Autodesk Fusion 360 part; units mm, degrees
note: some values were not read from the file. Set by a fixed rule: which sketch regions a step uses.
(part 2 of 5)
  line L811 (-126.9006, -75.4218) -> (-126.864, -75.6319)
  line L812 (-162.0421, -65.6576) -> (-162.1957, -65.5957)
  line L813 (-120.3905, -67.7689) -> (-120.173, -67.7759)
  line L814 (-90.103, -81.6973) -> (-90.112, -81.5125)
  line L815 (-65.5702, -65.5161) -> (-65.6778, -65.5555)
  line L816 (-93.5695, -76.6003) -> (-93.6281, -76.5038)
  line L817 (-126.8138, -65.8554) -> (-126.9169, -65.9479)
  line L818 (-87.0368, -78.1332) -> (-87.1608, -78.2349)
  line L819 (-140.2391, -65.691) -> (-140.3446, -65.6405)
  line L820 (-89.961, -66.5581) -> (-89.912, -66.407)
  line L821 (-115.4217, -76.295) -> (-115.4379, -76.172)
  line L822 (-129.347, -82.0733) -> (-129.353, -81.9536)
  line L823 (-50.3698, -71.3623) -> (-50.4116, -70.9586)
  line L824 (-93.7711, -77.986) -> (-93.6955, -77.9029)
  line L825 (-89.7734, -77.8951) -> (-89.8498, -77.7607)
  line L826 (-46.8782, -83.1526) -> (-46.7759, -83.1033)
  line L827 (-92.8846, -67.1853) -> (-92.9022, -67.0198)
  line L828 (-61.2627, -71.0913) -> (-61.2289, -70.9062)
  line L829 (-87.3025, -65.7007) -> (-87.1608, -65.7896)
  line L830 (-142.5953, -66.3913) -> (-142.6631, -66.5377)
  line L831 (-55.4106, -69.1495) -> (-55.2872, -69.243)
  line L832 (-103.1429, -65.6707) -> (-103.256, -65.7012)
  line L833 (-165.9299, -78.5695) -> (-165.7921, -78.5402)
  line L834 (-94.4542, -65.5719) -> (-94.5983, -65.5659)
  line L835 (-68.7045, -81.1031) -> (-68.801, -81.0445)
  line L836 (-169.2879, -78.2018) -> (-169.1558, -78.3005)
  line L837 (-123.2797, -75.1463) -> (-123.3556, -75.0225)
  line L838 (-76.8438, -76.0271) -> (-76.9461, -75.9778)
  line L839 (-55.8191, -68.9094) -> (-55.6766, -68.9828)
  line L840 (-62.1343, -82.9148) -> (-61.9869, -82.8077)
  line L841 (-80.9243, -80.5547) -> (-80.9006, -80.7493)
  line L842 (-121.6721, -67.9822) -> (-121.3798, -67.8915)
  line L843 (-76.9461, -75.9778) -> (-77.0536, -75.9384)
  line L844 (-163.1, -65.4919) -> (-163.2831, -65.5128)
  line L845 (-123.185, -75.2544) -> (-123.2797, -75.1463)
  line L846 (-101.2359, -66.5385) -> (-101.3094, -66.4135)
  line L847 (-120.0878, -75.693) -> (-120.2483, -75.693)
  line L848 (-116.4755, -75.1533) -> (-116.6326, -75.1503)
  line L849 (-87.0272, -82.7907) -> (-87.1556, -82.9073)
  line L850 (-53.6624, -82.7225) -> (-53.5344, -82.8302)
  line L851 (-121.4581, -71.9616) -> (-121.4203, -72.1465)
  line L852 (-133.3978, -83.1133) -> (-133.2339, -83.1617)
  line L853 (-132.6154, -83.2188) -> (-132.4975, -83.2377)
  line L854 (-141.2619, -78.1855) -> (-141.1327, -78.275)
  line L855 (-116.8006, -75.1659) -> (-120.0878, -75.693)
  line L856 (-169.912, -76.8783) -> (-169.903, -77.0537)
  line L857 (-123.4458, -74.7233) -> (-123.4576, -74.5459)
  line L858 (-121.3798, -67.8915) -> (-121.0683, -67.8246)
  line L859 (-120.6654, -78.2888) -> (-119.8307, -78.2988)
  line L860 (-119.8307, -78.2988) -> (-116.8014, -77.8018)
  line L861 (-134.2971, -66.4674) -> (-134.3507, -66.6361)
  line L862 (-111.0523, -65.5725) -> (-111.1974, -65.591)
  line L863 (-61.084, -70.3947) -> (-61.0214, -70.2386)
  line L864 (-130.9576, -67.0124) -> (-130.9813, -66.8178)
  line L865 (-142.5144, -66.252) -> (-142.5953, -66.3913)
  line L866 (-60.7916, -69.813) -> (-60.7012, -69.6851)
  line L867 (-59.2767, -68.7288) -> (-59.1098, -68.6816)
  line L868 (-94.7298, -65.5709) -> (-94.8598, -65.586)
  line L869 (-94.5986, -75.988) -> (-95.8873, -75.988)
  line L870 (-133.8257, -82.8864) -> (-133.6942, -82.9756)
  line L871 (-71.4648, -83.217) -> (-71.343, -83.2371)
  line L872 (-51.3135, -68.2591) -> (-51.4937, -67.9865)
  line L873 (-78.0556, -65.7513) -> (-78.1872, -65.6622)
  line L874 (-52.6036, -66.8344) -> (-52.8657, -66.6454)
  line L875 (-50.9966, -68.8468) -> (-51.1477, -68.5458)
  line L876 (-109.6365, -66.1302) -> (-109.7282, -66.0365)
  line L877 (-118.54, -68.7717) -> (-118.4981, -68.9082)
  line L878 (-59.8834, -68.9828) -> (-59.741, -68.9094)
  line L879 (-87.1608, -78.2349) -> (-87.3025, -78.3238)
  line L880 (-156.5375, -68.4558) -> (-156.4497, -68.5385)
  line L881 (-102.906, -65.6294) -> (-103.0505, -65.6498)
  line L882 (-89.4549, -82.9073) -> (-89.5832, -82.7907)
  line L883 (-61.5365, -82.243) -> (-61.4612, -82.0706)
  line L884 (-88.063, -78.5303) -> (-88.3059, -78.5393)
  line L885 (-90.037, -76.9765) -> (-90.042, -76.8042)
  line L886 (-141.3194, -65.4941) -> (-141.485, -65.5212)
  line L887 (-54.3644, -65.9031) -> (-54.7002, -65.7945)
  line L888 (-140.0758, -78.5266) -> (-139.8899, -78.489)
  line L889 (-110.6466, -65.5866) -> (-110.7765, -65.5715)
  line L890 (-126.9296, -74.973) -> (-126.9226, -75.2022)
  line L891 (-122.6439, -75.5491) -> (-122.801, -75.494)
  line L892 (-80.3369, -81.7452) -> (-80.2054, -81.8343)
  line L893 (-89.1489, -65.6257) -> (-88.9694, -65.5656)
  line L894 (-50.3366, -80.9037) -> (-50.3366, -72.2147)
  line L895 (-108.0032, -78.1266) -> (-107.8316, -78.1881)
  line L896 (-51.6881, -67.7282) -> (-51.8966, -67.4839)
  line L897 (-160.6206, -76.2253) -> (-160.7403, -76.2193)
  line L898 (-76.5741, -76.2287) -> (-76.6572, -76.1531)
  line L899 (-76.4986, -76.3118) -> (-76.5741, -76.2287)
  line L900 (-87.1556, -80.1182) -> (-87.0272, -80.2348)
  line L901 (-76.2839, -76.7083) -> (-76.3233, -76.6007)
  line L902 (-56.6229, -68.6408) -> (-56.4502, -68.6816)
  line L903 (-89.3159, -80.0143) -> (-89.1669, -79.9239)
  line L904 (-68.2121, -82.3098) -> (-68.1943, -82.1936)
  line L905 (-163.5051, -78.4641) -> (-163.3655, -78.4974)
  line L906 (-89.1669, -83.1019) -> (-89.3159, -83.0114)
  line L907 (-89.4507, -78.2349) -> (-89.5747, -78.1332)
  line L908 (-65.9667, -67.5363) -> (-65.8766, -67.6036)
  line L909 (-140.4165, -78.5316) -> (-140.2687, -78.5396)
  line L910 (-100.5686, -76.959) -> (-100.4851, -77.1166)
  line L911 (-111.7999, -65.8158) -> (-111.9405, -65.911)
  line L912 (-52.9126, -83.1337) -> (-52.7317, -83.1755)
  line L913 (-141.6874, -76.173) -> (-141.7635, -76.2923)
  line L914 (-95.4672, -65.8024) -> (-95.5765, -65.8721)
  line L915 (-77.8284, -65.9697) -> (-77.9359, -65.8538)
  line L916 (-86.9295, -66.005) -> (-86.8381, -66.1295)
  line L917 (-77.7337, -66.0989) -> (-77.8284, -65.9697)
  line L918 (-46.3046, -81.516) -> (-46.3632, -81.4195)
  line L919 (-87.941, -79.7427) -> (-87.7677, -79.7872)
  line L920 (-129.4881, -82.6312) -> (-129.4388, -82.5289)
  line L921 (-81.9787, -75.9472) -> (-82.1648, -75.9512)
  line L922 (-80.9323, -69.0045) -> (-80.9323, -75.9472)
  line L923 (-164.0956, -78.1584) -> (-163.9927, -78.2379)
  line L924 (-80.9323, -68.559) -> (-80.9323, -69.0045)
  line L925 (-77.1657, -78.2028) -> (-77.0536, -78.1739)
  line L926 (-108.6242, -77.7613) -> (-108.4802, -77.8696)
  line L927 (-93.6955, -77.9029) -> (-93.6281, -77.8128)
  line L928 (-89.8498, -66.2638) -> (-89.7734, -66.1295)
  line L929 (-102.7483, -65.6214) -> (-102.7533, -65.6214)
  line L930 (-77.2819, -78.2205) -> (-77.1657, -78.2028)
  line L931 (-77.4016, -78.2265) -> (-77.2819, -78.2205)
  line L932 (-88.3054, -79.7063) -> (-88.1205, -79.7153)
  line L933 (-52.3545, -67.0371) -> (-52.6036, -66.8344)
  line L934 (-72.1359, -83.085) -> (-71.9818, -83.1371)
  line L935 (-142.7171, -66.6901) -> (-142.7566, -66.8474)
  line L936 (-116.0697, -75.2646) -> (-116.1941, -75.2121)
  line L937 (-121.0683, -67.8246) -> (-120.7384, -67.7832)
  line L938 (-86.5074, -81.6973) -> (-86.5348, -81.8768)
  line L939 (-46.2553, -81.6183) -> (-46.3046, -81.516)
  line L940 (-78.1872, -65.6622) -> (-78.33, -65.5866)
  line L941 (-80.9323, -67.1493) -> (-80.9323, -68.559)
  line L942 (-68.4557, -82.8183) -> (-68.3883, -82.7282)
  line L943 (-77.6522, -66.2413) -> (-77.7337, -66.0989)
  line L944 (-106.2087, -78.1313) -> (-106.0461, -78.0602)
  line L945 (-61.8395, -66.1717) -> (-62.1152, -66.3088)
  line L946 (-69.632, -67.0129) -> (-69.6557, -66.8183)
  line L947 (-68.3883, -82.7282) -> (-68.3296, -82.6317)
  line L948 (-102.1409, -65.739) -> (-102.2516, -65.7009)
  line L949 (-141.3833, -78.0849) -> (-141.2619, -78.1855)
  line L950 (-62.9317, -66.2857) -> (-62.9711, -66.1782)
  line L951 (-106.5499, -78.2376) -> (-106.3768, -78.1906)
  line L952 (-160.2848, -78.4671) -> (-160.1826, -78.4179)
  line L953 (-160.5044, -76.243) -> (-160.6206, -76.2253)
  line L954 (-82.7955, -76.0449) -> (-82.9243, -76.0896)
  line L955 (-160.3923, -76.2718) -> (-160.5044, -76.243)
  line L956 (-164.4833, -77.6255) -> (-164.4235, -77.7499)
  line L957 (-54.237, -71.9056) -> (-54.237, -81.2746)
  line L958 (-160.3923, -78.5064) -> (-160.2848, -78.4671)
  line L959 (-82.9243, -76.0896) -> (-83.0413, -76.1434)
  line L960 (-160.2848, -76.3111) -> (-160.3923, -76.2718)
  line L961 (-130.3974, -80.9088) -> (-130.5171, -80.9028)
  line L962 (-112.6217, -67.1857) -> (-112.6227, -67.3536)
  line L963 (-86.8066, -80.5021) -> (-86.7161, -80.6511)
  line L964 (-54.241, -71.6908) -> (-54.237, -71.9056)
  line L965 (-90.0756, -81.1482) -> (-90.0311, -80.975)
  line L966 (-60.9517, -65.8277) -> (-61.2576, -65.9312)
  line L967 (-87.6422, -65.5656) -> (-87.4627, -65.6257)
  line L968 (-77.5844, -81.0996) -> (-77.5308, -80.931)
  line L969 (-77.7337, -81.3976) -> (-77.6522, -81.2552)
  line L970 (-130.1691, -80.9553) -> (-130.2812, -80.9265)
  line L971 (-110.908, -65.5665) -> (-111.0523, -65.5725)
  line L972 (-66.3009, -67.089) -> (-66.2516, -67.1913)
  line L973 (-77.9359, -65.8538) -> (-78.0556, -65.7513)
  line L974 (-77.4602, -68.559) -> (-77.4602, -67.1493)
  line L975 (-160.0861, -78.3594) -> (-159.996, -78.2921)
  line L976 (-132.8771, -83.2173) -> (-132.6852, -83.2248)
  line L977 (-93.5666, -65.9106) -> (-93.7072, -65.8154)
  line L978 (-63.6988, -83.1888) -> (-63.4915, -83.2157)
  line L979 (-140.4577, -65.5959) -> (-140.5788, -65.5579)
  line L980 (-65.2215, -71.648) -> (-65.207, -71.7916)
  line L981 (-92.9826, -67.8593) -> (-92.9319, -67.6912)
  line L982 (-69.816, -66.3124) -> (-69.8975, -66.17)
  line L983 (-89.309, -65.7007) -> (-89.1489, -65.6257)
  line L984 (-46.1692, -82.1938) -> (-46.1632, -82.0741)
  line L985 (-94.479, -75.994) -> (-94.5986, -75.988)
  line L986 (-66.1255, -65.8894) -> (-66.1929, -65.9795)
  line L987 (-46.187, -81.8381) -> (-46.2159, -81.7259)
  line L988 (-94.1431, -76.0799) -> (-94.2506, -76.0405)
  line L989 (-133.9455, -65.9244) -> (-134.053, -66.0402)
  line L990 (-88.3059, -65.4852) -> (-88.063, -65.4942)
  line L991 (-140.8562, -78.4181) -> (-140.7116, -78.4701)
  line L992 (-135.39, -73.3534) -> (-135.3726, -73.1817)
  line L993 (-68.6144, -81.1705) -> (-68.7045, -81.1031)
  line L994 (-142.6631, -66.5377) -> (-142.7171, -66.6901)
  line L995 (-131.3176, -66.0402) -> (-131.425, -65.9244)
  line L996 (-141.9093, -76.9708) -> (-141.8993, -77.1333)
  line L997 (-69.6557, -66.8183) -> (-69.6946, -66.6366)
  line L998 (-106.0461, -78.0602) -> (-105.8898, -77.9776)
  line L999 (-50.7395, -69.4922) -> (-50.8605, -69.1623)
  line L1000 (-129.9593, -83.1025) -> (-129.8628, -83.0439)
  line L1001 (-134.053, -82.6678) -> (-133.9455, -82.7838)
  line L1002 (-50.6339, -69.8368) -> (-50.7395, -69.4922)
  line L1003 (-77.1657, -75.9096) -> (-77.2819, -75.8919)
  line L1004 (-129.6141, -82.8178) -> (-129.5467, -82.7277)
  line L1005 (-105.4645, -77.6658) -> (-105.3395, -77.542)
  line L1006 (-93.8589, -65.7335) -> (-94.0212, -65.666)
  line L1007 (-89.7734, -66.1295) -> (-89.682, -66.005)
  line L1008 (-54.1178, -82.0155) -> (-54.0527, -82.1779)
  line L1009 (-86.6505, -77.4665) -> (-86.6995, -77.6175)
  line L1010 (-107.6547, -78.2368) -> (-107.4733, -78.2722)
  line L1011 (-80.9006, -80.7493) -> (-80.8617, -80.931)
  line L1012 (-63.3951, -65.6634) -> (-63.4916, -65.6048)
  line L1013 (-61.5536, -66.0458) -> (-61.8395, -66.1717)
  line L1014 (-80.8081, -66.3968) -> (-80.8617, -66.5655)
  line L1015 (-131.819, -65.6573) -> (-131.9726, -65.5954)
  line L1016 (-65.1882, -81.6928) -> (-65.1452, -81.887)
  line L1017 (-89.682, -66.005) -> (-89.5747, -65.8914)
  line L1018 (-131.2229, -66.1694) -> (-131.3176, -66.0402)
  line L1019 (-82.3396, -78.2162) -> (-82.1648, -78.2274)
  line L1020 (-82.6551, -76.009) -> (-82.7955, -76.0449)
  line L1021 (-160.7403, -78.5589) -> (-160.6206, -78.5529)
  line L1022 (-165.2902, -78.3193) -> (-165.1793, -78.2406)
  line L1023 (-164.5745, -77.3505) -> (-164.5337, -77.4924)
  line L1024 (-160.6206, -78.5529) -> (-160.5044, -78.5352)
  line L1025 (-163.6379, -78.4215) -> (-163.5051, -78.4641)
  line L1026 (-102.0887, -65.7551) -> (-102.1409, -65.739)
  line L1027 (-129.4388, -82.5289) -> (-129.3995, -82.4213)
  line L1028 (-78.1873, -81.8343) -> (-78.0558, -81.7452)
  line L1029 (-79.1963, -65.4138) -> (-79.3881, -65.4208)
  line L1030 (-79.3881, -65.4208) -> (-79.5712, -65.4417)
  line L1031 (-80.0624, -65.5866) -> (-80.2052, -65.6622)
  line L1032 (-77.0536, -78.1739) -> (-76.9461, -78.1345)
  line L1033 (-76.9461, -78.1345) -> (-76.8438, -78.0852)
  line L1034 (-80.4566, -81.6427) -> (-80.3369, -81.7452)
  line L1035 (-87.0368, -65.8914) -> (-86.9295, -66.005)
  line L1036 (-82.7955, -78.134) -> (-82.6551, -78.1698)
  line L1037 (-77.2819, -75.8919) -> (-77.4016, -75.8859)
  line L1038 (-142.4321, -68.291) -> (-138.8179, -73.1413)
  line L1039 (-133.0602, -65.5125) -> (-133.2339, -65.5471)
  line L1040 (-63.8136, -65.4873) -> (-63.9298, -65.4696)
  line L1041 (-117.4702, -65.7305) -> (-117.6443, -65.6736)
  line L1042 (-78.6478, -82.0202) -> (-78.4838, -81.9719)
  line L1043 (-66.3928, -66.6336) -> (-66.3868, -66.7532)
  line L1044 (-53.4283, -66.3082) -> (-53.7283, -66.1599)
  line L1045 (-93.6281, -77.8128) -> (-93.5695, -77.7163)
  line L1046 (-68.2409, -82.4219) -> (-68.2121, -82.3098)
  line L1047 (-139.3769, -78.2514) -> (-139.2218, -78.1381)
  line L1048 (-76.3726, -76.4984) -> (-76.4312, -76.4019)
  line L1049 (-142.5381, -68.1262) -> (-142.4321, -68.291)
  line L1050 (-86.5888, -66.8796) -> (-86.5744, -67.0481)
  line L1051 (-86.9106, -80.3631) -> (-86.8066, -80.5021)
  line L1052 (-78.33, -65.5866) -> (-78.4836, -65.5246)
  line L1053 (-89.1669, -79.9239) -> (-89.0089, -79.8479)
  line L1054 (-52.1188, -67.2535) -> (-52.3545, -67.0371)
  line L1055 (-92.8991, -67.5221) -> (-92.8836, -67.3531)
  line L1056 (-78.4836, -65.5246) -> (-78.6475, -65.4763)
  line L1057 (-78.6475, -65.4763) -> (-78.8213, -65.4417)
  line L1058 (-77.5308, -66.5655) -> (-77.5844, -66.3968)
  line L1059 (-65.3418, -65.4696) -> (-65.458, -65.4873)
  line L1060 (-77.5844, -66.3968) -> (-77.6522, -66.2413)
  line L1061 (-100.6403, -76.7941) -> (-100.5686, -76.959)
  line L1062 (-61.1395, -70.5579) -> (-61.084, -70.3947)
  line L1063 (-87.6422, -78.4589) -> (-87.842, -78.5031)
  line L1064 (-71.6462, -83.2032) -> (-71.4648, -83.217)
  line L1065 (-94.1649, -65.6216) -> (-94.3095, -65.5904)
  line L1066 (-65.207, -71.7916) -> (-65.2174, -72.0012)
  line L1067 (-140.708, -65.5271) -> (-140.8458, -65.5044)
  line L1068 (-131.9726, -65.5954) -> (-132.1365, -65.5471)
  line L1069 (-134.2971, -82.2404) -> (-134.2293, -82.396)
  line L1070 (-108.8856, -77.5138) -> (-108.7595, -77.6426)
  line L1071 (-64.5603, -82.8077) -> (-64.4129, -82.9148)
  line L1072 (-61.9869, -82.8077) -> (-61.8529, -82.6864)
  line L1073 (-93.4342, -77.2781) -> (-93.4282, -77.1585)
  line L1074 (-89.4507, -65.7896) -> (-89.309, -65.7007)
  line L1075 (-50.8605, -69.1623) -> (-50.9966, -68.8468)
  line L1076 (-77.4602, -78.2305) -> (-77.4602, -78.2265)
  line L1077 (-87.1556, -82.9073) -> (-87.2947, -83.0114)
  line L1078 (-56.4502, -68.6816) -> (-56.2833, -68.7288)
  line L1079 (-66.3691, -66.8694) -> (-66.3403, -66.9815)
  line L1080 (-141.5971, -77.8536) -> (-141.4955, -77.9741)
  line L1081 (-63.2219, -65.8063) -> (-63.305, -65.7308)
  line L1082 (-79.0043, -65.4208) -> (-79.1963, -65.4138)
  line L1083 (-76.6572, -76.1531) -> (-76.7473, -76.0857)
  line L1084 (-80.2052, -65.6622) -> (-80.3368, -65.7513)
  line L1085 (-100.045, -77.6636) -> (-99.9116, -77.7774)
  line L1086 (-76.7473, -78.0266) -> (-76.6572, -77.9592)
  line L1087 (-77.4919, -80.7493) -> (-77.4682, -80.5547)
  line L1088 (-63.1464, -65.8894) -> (-63.2219, -65.8063)
  line L1089 (-77.4602, -67.1493) -> (-77.4682, -66.9418)
  line L1090 (-78.0558, -81.7452) -> (-77.936, -81.6427)
  line L1091 (-92.9319, -67.6912) -> (-92.8991, -67.5221)
  line L1092 (-108.169, -78.0527) -> (-108.0032, -78.1266)
  line L1093 (-70.9852, -65.5129) -> (-71.1683, -65.492)
  line L1094 (-46.187, -82.31) -> (-46.1692, -82.1938)
  line L1095 (-65.2144, -81.4884) -> (-65.1882, -81.6928)
  line L1096 (-141.8708, -76.5779) -> (-141.8993, -76.7576)
  line L1097 (-99.1359, -78.1876) -> (-98.9634, -78.2348)
  line L1098 (-68.5313, -82.9014) -> (-68.4557, -82.8183)
  line L1099 (-134.4213, -73.5926) -> (-134.4213, -81.4877)
  line L1100 (-164.6721, -77.6095) -> (-164.6183, -77.4824)
  line L1101 (-81.9787, -78.2305) -> (-80.9323, -78.2305)
  line L1102 (-164.1904, -78.0698) -> (-164.0956, -78.1584)
  line L1103 (-66.3403, -66.9815) -> (-66.3009, -67.089)
  line L1104 (-69.3591, -83.2441) -> (-69.2394, -83.2381)
  line L1105 (-132.8771, -65.4916) -> (-133.0602, -65.5125)
  line L1106 (-51.4937, -67.9865) -> (-51.6881, -67.7282)
  line L1107 (-79.7449, -65.4763) -> (-79.9088, -65.5246)
  line L1108 (-52.8657, -66.6454) -> (-53.1407, -66.4701)
  line L1109 (-86.64, -80.809) -> (-86.5793, -80.975)
  line L1110 (-66.1929, -65.9795) -> (-66.2516, -66.076)
  line L1111 (-65.6778, -65.5555) -> (-65.7801, -65.6048)
  line L1112 (-66.0499, -65.8063) -> (-66.1255, -65.8894)
  line L1113 (-58.167, -65.3954) -> (-58.5464, -65.4115)
  line L1114 (-69.3591, -80.9033) -> (-69.624, -80.9033)
  line L1115 (-77.4682, -66.9418) -> (-77.4919, -66.7472)
  line L1116 (-80.7403, -66.2413) -> (-80.8081, -66.3968)
  line L1117 (-140.997, -78.3528) -> (-140.8562, -78.4181)
  line L1118 (-106.3768, -78.1906) -> (-106.2087, -78.1313)
  line L1119 (-166.4853, -75.6143) -> (-168.1963, -75.6143)
  line L1120 (-123.3556, -75.0225) -> (-123.4114, -74.8818)
  line L1121 (-86.5744, -76.9765) -> (-86.5888, -77.145)
  line L1122 (-77.4602, -78.2265) -> (-77.4016, -78.2265)
  line L1123 (-73.089, -81.689) -> (-73.0668, -81.8773)
  line L1124 (-71.7351, -65.5129) -> (-71.9088, -65.5475)
  line L1125 (-94.5983, -65.5659) -> (-94.7298, -65.5709)
  line L1126 (-169.5204, -77.9693) -> (-169.4097, -78.0911)
  line L1127 (-89.5832, -80.2348) -> (-89.4549, -80.1182)
  line L1128 (-141.825, -77.4421) -> (-141.7632, -77.5869)
  line L1129 (-68.2803, -81.618) -> (-68.3296, -81.5157)
  line L1130 (-80.0626, -81.9099) -> (-79.909, -81.9719)
  line L1131 (-59.9762, -65.5837) -> (-60.3108, -65.654)
  line L1132 (-63.9298, -65.4696) -> (-64.0494, -65.4636)
  line L1133 (-88.4902, -83.3107) -> (-88.6697, -83.2833)
  line L1134 (-62.6352, -66.6169) -> (-62.8792, -66.7881)
  line L1135 (-77.6522, -81.2552) -> (-77.5844, -81.0996)
  line L1136 (-88.6697, -79.7427) -> (-88.4902, -79.7153)
  line L1137 (-71.8185, -83.1765) -> (-71.6462, -83.2032)
  line L1138 (-141.6868, -77.7243) -> (-141.5971, -77.8536)
  line L1139 (-90.042, -67.2203) -> (-90.037, -67.0481)
  line L1140 (-131.5448, -65.8219) -> (-131.6763, -65.7328)
  line L1141 (-53.395, -82.9256) -> (-53.2446, -83.0083)
  line L1142 (-141.485, -65.5212) -> (-141.644, -65.5652)
  line L1143 (-134.053, -66.0402) -> (-134.1478, -66.1694)
  line L1144 (-136.2972, -70.9305) -> (-139.5794, -66.2933)
  line L1145 (-54.229, -81.4727) -> (-54.2064, -81.6625)
  line L1146 (-96.1018, -66.4544) -> (-96.1626, -66.5764)
  line L1147 (-123.4114, -74.8818) -> (-123.4458, -74.7233)
  line L1148 (-53.7283, -66.1599) -> (-54.0404, -66.0248)
  line L1149 (-121.0588, -72.7204) -> (-120.9345, -72.8083)
  line L1150 (-71.2172, -83.2441) -> (-69.3591, -83.2441)
  line L1151 (-101.5617, -66.1074) -> (-101.65, -66.0281)
  line L1152 (-139.965, -65.8704) -> (-140.1409, -65.7466)
  line L1153 (-135.4061, -72.608) -> (-135.4516, -72.4184)
  line L1154 (-80.9323, -75.9472) -> (-81.9787, -75.9472)
  line L1155 (-141.9397, -65.6991) -> (-142.0749, -65.7869)
  line L1156 (-107.0214, -73.0608) -> (-109.2926, -66.7055)
  line L1157 (-93.5202, -76.7026) -> (-93.5695, -76.6003)
  line L1158 (-72.6504, -82.7506) -> (-72.538, -82.853)
  line L1159 (-65.9667, -65.7308) -> (-66.0499, -65.8063)
  line L1160 (-93.7072, -65.8154) -> (-93.8589, -65.7335)
  line L1161 (-132.1365, -65.5471) -> (-132.3103, -65.5125)
  line L1162 (-112.1863, -66.137) -> (-112.2905, -66.2655)
  line L1163 (-61.3325, -81.4884) -> (-61.3235, -81.2746)
  line L1164 (-64.8142, -82.5514) -> (-64.6942, -82.6864)
  line L1165 (-72.9802, -82.2175) -> (-72.9166, -82.3692)
  line L1166 (-140.7116, -78.4701) -> (-140.5646, -78.5082)
  line L1167 (-86.9295, -78.0196) -> (-87.0368, -78.1332)
  line L1168 (-133.8257, -65.8219) -> (-133.9455, -65.9244)
  line L1169 (-61.2289, -70.9062) -> (-61.1878, -70.7284)
  line L1170 (-86.5694, -67.2203) -> (-86.5694, -76.8042)
  line L1171 (-69.1231, -80.927) -> (-69.2394, -80.9093)
  line L1172 (-72.904, -66.3124) -> (-72.9718, -66.468)
  line L1173 (-89.1489, -78.3988) -> (-89.309, -78.3238)
  line L1174 (-135.641, -74.1334) -> (-135.54, -73.9208)
  line L1175 (-133.5514, -83.0512) -> (-133.3978, -83.1133)
  line L1176 (-72.3691, -65.7333) -> (-72.5006, -65.8224)
  line L1177 (-65.0105, -82.243) -> (-64.9198, -82.4034)
  line L1178 (-98.9634, -78.2348) -> (-98.7865, -78.2694)
  line L1179 (-52.2486, -83.2445) -> (-47.3337, -83.2445)
  line L1180 (-120.8032, -72.878) -> (-120.6684, -72.9315)
  line L1181 (-72.4145, -82.9429) -> (-72.2803, -83.0202)
  line L1182 (-111.1974, -65.591) -> (-111.3423, -65.6222)
  line L1183 (-121.1729, -72.6123) -> (-121.0588, -72.7204)
  line L1184 (-76.2374, -77.1762) -> (-76.2314, -77.0566)
  line L1185 (-63.079, -65.9795) -> (-63.1464, -65.8894)
  line L1186 (-63.0204, -66.076) -> (-63.079, -65.9795)
  line L1187 (-46.6794, -81.1034) -> (-46.7759, -81.0448)
  line L1188 (-102.7551, -65.6214) -> (-102.7591, -65.6214)
  line L1189 (-70.8115, -65.5475) -> (-70.9852, -65.5129)
  line L1190 (-159.8374, -76.6449) -> (-159.9129, -76.5618)
  line L1191 (-68.6144, -82.9769) -> (-68.5313, -82.9014)
  line L1192 (-83.3896, -76.4563) -> (-83.4462, -76.5605)
  line L1193 (-82.1648, -75.9512) -> (-82.3396, -75.9626)
  line L1194 (-82.3396, -75.9626) -> (-82.5031, -75.9816)
  line L1195 (-131.6763, -65.7328) -> (-131.819, -65.6573)
  line L1196 (-129.8628, -83.0439) -> (-129.7727, -82.9765)
  line L1197 (-165.7921, -78.5402) -> (-165.6589, -78.5)
  line L1198 (-82.5031, -75.9816) -> (-82.6551, -76.009)
  line L1199 (-123.4038, -69.8118) -> (-123.3375, -69.5795)
  line L1200 (-93.5695, -77.7163) -> (-93.5202, -77.614)
  line L1201 (-138.8179, -73.1413) -> (-141.3861, -75.8284)
  line L1202 (-76.4312, -76.4019) -> (-76.4986, -76.3118)
  line L1203 (-115.8534, -75.4086) -> (-115.9561, -75.3306)
  line L1204 (-135.3666, -72.9978) -> (-135.3769, -72.8016)
  line L1205 (-139.6868, -66.1494) -> (-139.8145, -66.0066)
  line L1206 (-118.4726, -69.384) -> (-118.5, -69.5598)
  line L1207 (-62.3805, -66.4572) -> (-62.6352, -66.6169)
  line L1208 (-62.8792, -66.7881) -> (-62.8792, -66.6336)
  line L1209 (-63.5939, -65.5555) -> (-63.7014, -65.5161)
  line L1210 (-130.2812, -83.22) -> (-130.1691, -83.1912)
  line L1211 (-63.4916, -65.6048) -> (-63.5939, -65.5555)
  line L1212 (-162.5987, -78.5589) -> (-160.7403, -78.5589)
  line L1213 (-68.2803, -82.5294) -> (-68.2409, -82.4219)
  line L1214 (-162.72, -78.5529) -> (-162.5987, -78.5589)
  line L1215 (-159.996, -76.4863) -> (-160.0861, -76.419)
  line L1216 (-76.2374, -76.9369) -> (-76.2551, -76.8206)
  line L1217 (-68.3296, -81.5157) -> (-68.3883, -81.4192)
  line L1218 (-83.2396, -76.2797) -> (-83.3207, -76.3628)
  line L1219 (-69.9923, -66.0408) -> (-70.0998, -65.9249)
  line L1220 (-96.2143, -66.7049) -> (-98.4858, -73.0619)
  line L1221 (-71.9088, -65.5475) -> (-72.0727, -65.5958)
  line L1222 (-88.8429, -79.7872) -> (-88.6697, -79.7427)
  line L1223 (-159.7115, -76.8314) -> (-159.7701, -76.7349)
  line L1224 (-134.1478, -66.1694) -> (-134.2293, -66.3118)
  line L1225 (-83.4904, -76.6757) -> (-83.5221, -76.8021)
  line L1226 (-58.937, -68.6408) -> (-58.574, -68.5784)
  line L1227 (-101.65, -66.0281) -> (-101.743, -65.9554)
  line L1228 (-164.5337, -77.4924) -> (-164.4833, -77.6255)
  line L1229 (-159.7701, -76.7349) -> (-159.8374, -76.6449)
  line L1230 (-147.3075, -77.2905) -> (-147.0665, -77.0991)
  line L1231 (-78.4838, -81.9719) -> (-78.3302, -81.9099)
  line L1232 (-86.4984, -81.5125) -> (-86.5074, -81.6973)
  line L1233 (-83.4462, -76.5605) -> (-83.4904, -76.6757)
  line L1234 (-71.1683, -65.492) -> (-71.3602, -65.485)
  line L1235 (-139.8145, -66.0066) -> (-139.965, -65.8704)
  line L1236 (-76.5741, -77.8837) -> (-76.4986, -77.8006)
  line L1237 (-87.7677, -83.2388) -> (-87.941, -83.2833)
  line L1238 (-61.0214, -70.2386) -> (-60.9517, -70.0896)
  line L1239 (-139.5794, -66.2933) -> (-139.6868, -66.1494)
  line L1240 (-129.353, -81.9536) -> (-129.3707, -81.8373)
  line L1241 (-139.8899, -78.489) -> (-139.7112, -78.4291)
  line L1242 (-77.4919, -66.7472) -> (-77.5308, -66.5655)
  line L1243 (-54.539, -70.2386) -> (-54.4764, -70.3947)
  line L1244 (-57.3718, -68.5413) -> (-56.986, -68.5784)
  line L1245 (-46.5893, -81.1708) -> (-46.6794, -81.1034)
  line L1246 (-55.0473, -65.699) -> (-55.4058, -65.6166)
  line L1247 (-76.2314, -77.0566) -> (-76.2374, -76.9369)
  line L1248 (-93.4375, -66.0181) -> (-93.5666, -65.9106)
  line L1249 (-88.1205, -83.3107) -> (-88.3054, -83.3197)
  line L1250 (-77.4602, -80.3472) -> (-77.4602, -78.2305)
  line L1251 (-104.3427, -66.6878) -> (-107.0214, -73.0608)
  line L1252 (-53.1407, -66.4701) -> (-53.4283, -66.3082)
  line L1253 (-107.4733, -78.2722) -> (-107.288, -78.2938)
  line L1254 (-163.7636, -78.3695) -> (-163.6379, -78.4215)
  line L1255 (-63.7014, -65.5161) -> (-63.8136, -65.4873)
  line L1256 (-69.1231, -83.2204) -> (-69.0109, -83.1916)
  line L1257 (-119.8428, -73.0222) -> (-119.3494, -72.958)
  line L1258 (-163.882, -78.3083) -> (-163.7636, -78.3695)
  line L1259 (-87.6017, -79.8479) -> (-87.4437, -79.9239)
  line L1260 (-160.0861, -76.419) -> (-160.1826, -76.3604)
  line L1261 (-83.0413, -76.1434) -> (-83.1465, -76.2067)
  line L1262 (-70.3511, -65.7333) -> (-70.4939, -65.6578)
  line L1263 (-160.1826, -76.3604) -> (-160.2848, -76.3111)
  line L1264 (-66.3868, -66.514) -> (-66.3928, -66.6336)
  line L1265 (-95.2348, -65.6887) -> (-95.3531, -65.7412)
  line L1266 (-70.6475, -65.5958) -> (-70.8115, -65.5475)
  line L1267 (-159.9129, -76.5618) -> (-159.996, -76.4863)
  line L1268 (-83.3896, -77.7235) -> (-83.3207, -77.8168)
  line L1269 (-133.2339, -65.5471) -> (-133.3978, -65.5954)
  line L1270 (-83.1465, -76.2067) -> (-83.2396, -76.2797)
  line L1271 (-86.6139, -66.7159) -> (-86.5888, -66.8796)
  line L1272 (-163.3655, -78.4974) -> (-163.2193, -78.5212)
  line L1273 (-83.3207, -76.3628) -> (-83.3896, -76.4563)
  line L1274 (-98.3201, -78.293) -> (-98.1858, -78.3189)
  line L1275 (-112.5246, -67.8603) -> (-109.3525, -76.7362)
  line L1276 (-164.8891, -77.9561) -> (-164.808, -77.8468)
  line L1277 (-141.3861, -75.8284) -> (-141.5982, -76.0604)
  line L1278 (-150.0636, -68.4918) -> (-149.9234, -68.559)
  line L1279 (-105.2238, -77.4089) -> (-105.1182, -77.267)
  line L1280 (-161.6481, -65.9247) -> (-161.7678, -65.8222)
  line L1281 (-64.6942, -82.6864) -> (-64.5603, -82.8077)
  line L1282 (-102.7533, -65.6214) -> (-102.7543, -65.6214)
  line L1283 (-59.2792, -65.4759) -> (-59.6322, -65.5243)
  line L1284 (-72.8402, -82.5087) -> (-72.7513, -82.6359)
  line L1285 (-80.6588, -66.0989) -> (-80.7403, -66.2413)
  line L1286 (-110.5188, -65.6115) -> (-110.6466, -65.5866)
  line L1287 (-68.3296, -82.6317) -> (-68.2803, -82.5294)
  line L1288 (-168.1962, -78.5935) -> (-166.2167, -78.5935)
  line L1289 (-89.8038, -82.5231) -> (-89.8943, -82.3741)
  line L1290 (-86.9106, -82.6623) -> (-87.0272, -82.7907)
  line L1291 (-89.682, -78.0196) -> (-89.7734, -77.8951)
  line L1292 (-99.9116, -77.7774) -> (-99.7701, -77.8812)
  line L1293 (-68.2121, -81.8379) -> (-68.2409, -81.7256)
  line L1294 (-46.4306, -82.8186) -> (-46.3632, -82.7285)
  line L1295 (-95.6805, -65.95) -> (-95.7786, -66.0359)
  line L1296 (-93.2162, -66.2652) -> (-93.3205, -66.1366)
  line L1297 (-60.0196, -69.0628) -> (-59.8834, -68.9828)
  line L1298 (-101.3514, -66.355) -> (-101.4211, -66.2621)
  line L1299 (-82.6551, -78.1698) -> (-82.5031, -78.1971)
  line L1300 (-70.0998, -65.9249) -> (-70.2196, -65.8224)
  line L1301 (-71.3602, -65.485) -> (-71.5521, -65.492)
  line L1302 (-58.9172, -65.4383) -> (-59.2792, -65.4759)
  line L1303 (-103.0505, -65.6498) -> (-103.1429, -65.6707)
  line L1304 (-115.0478, -69.7836) -> (-115.0167, -69.5432)
  line L1305 (-146.032, -67.9697) -> (-146.2105, -67.7326)
  line L1306 (-115.0907, -70.0127) -> (-115.0478, -69.7836)
  line L1307 (-127.213, -66.401) -> (-127.2532, -66.5328)
  line L1308 (-116.9672, -65.9437) -> (-117.1313, -65.8656)
  line L1309 (-121.2734, -72.482) -> (-121.1729, -72.6123)
  line L1310 (-118.6087, -69.8735) -> (-118.6897, -70.0123)
  line L1311 (-157.3044, -71.5845) -> (-157.3994, -71.6624)
  line L1312 (-116.6513, -66.1205) -> (-116.8071, -66.0287)
  line L1313 (-126.9849, -68.2467) -> (-126.9621, -68.439)
  line L1314 (-126.9169, -65.9479) -> (-127.0093, -66.0492)
  line L1315 (-118.7882, -70.1398) -> (-118.9041, -70.2565)
  line L1316 (-156.6012, -71.3747) -> (-156.7744, -71.3956)
  line L1317 (-115.0145, -68.6272) -> (-115.0419, -68.4346)
  line L1318 (-141.4955, -77.9741) -> (-141.3833, -78.0849)
  line L1319 (-121.0036, -71.031) -> (-121.0851, -71.081)
  line L1320 (-120.0568, -73.0282) -> (-119.9037, -73.0252)
  line L1321 (-115.185, -67.8882) -> (-115.2518, -67.7168)
  line L1322 (-115.0797, -68.2472) -> (-115.1275, -68.065)
  line L1323 (-121.1665, -71.1421) -> (-121.2446, -71.2152)
  line L1324 (-146.8308, -67.0731) -> (-147.0666, -66.8727)
  line L1325 (-117.1373, -72.3811) -> (-116.9469, -72.2931)
  line L1326 (-115.3749, -70.8221) -> (-115.2876, -70.6352)
  line L1327 (-116.7634, -72.1984) -> (-116.5871, -72.0968)
  line L1328 (-122.6149, -66.5573) -> (-122.887, -66.7624)
  line L1329 (-153.8149, -78.1635) -> (-153.5078, -78.2604)
  line L1330 (-157.7056, -72.4512) -> (-157.7189, -72.6442)
  line L1331 (-58.574, -68.5784) -> (-58.1882, -68.5413)
  line L1332 (-120.5332, -72.9709) -> (-120.4012, -72.9983)
  line L1333 (-122.3375, -66.3725) -> (-122.6149, -66.5573)
  line L1334 (-124.1506, -66.0932) -> (-124.2785, -65.9603)
  line L1335 (-118.916, -65.4843) -> (-119.2563, -65.4903)
  line L1336 (-124.0398, -66.2386) -> (-124.1506, -66.0932)
  line L1337 (-125.7165, -65.4841) -> (-125.8714, -65.4901)
  line L1338 (-157.696, -73.3909) -> (-157.6629, -73.6565)
  line L1339 (-117.9999, -65.5818) -> (-118.1807, -65.547)
  line L1340 (-157.4856, -74.441) -> (-157.4009, -74.6967)
  line L1341 (-152.1737, -78.5079) -> (-151.8143, -78.5322)
  line L1342 (-119.9539, -70.7594) -> (-120.1863, -70.8151)
  line L1343 (-148.0994, -77.7881) -> (-147.824, -77.6353)
  line L1344 (-157.6826, -72.2773) -> (-157.7056, -72.4512)
  line L1345 (-157.7229, -72.8568) -> (-157.7159, -73.1242)
  line L1346 (-153.5078, -78.2604) -> (-153.19, -78.3438)
  line L1347 (-156.7897, -75.9092) -> (-156.6307, -76.1348)
  line L1348 (-156.6307, -76.1348) -> (-156.4597, -76.3536)
  line L1349 (-154.3968, -77.9313) -> (-154.1113, -78.0537)
  line L1350 (-154.1113, -78.0537) -> (-153.8149, -78.1635)
  line L1351 (-146.8374, -76.8954) -> (-146.6201, -76.6795)
  line L1352 (-146.6201, -76.6795) -> (-146.4149, -76.4518)
  line L1353 (-157.7189, -72.6442) -> (-157.7229, -72.8568)
  line L1354 (-151.064, -78.5322) -> (-150.6931, -78.5087)
  line L1355 (-157.0712, -75.4395) -> (-156.9366, -75.6773)
  line L1356 (-157.7159, -73.1242) -> (-157.696, -73.3909)
  line L1357 (-151.8143, -78.5322) -> (-151.4448, -78.5402)
  line L1358 (-157.5576, -74.182) -> (-157.4856, -74.441)
  line L1359 (-153.19, -78.3438) -> (-152.8617, -78.4132)
  line L1360 (-156.4597, -76.3536) -> (-156.2767, -76.5651)
  line L1361 (-144.93, -70.9336) -> (-144.9689, -70.6491)
  line L1362 (-150.6931, -78.5087) -> (-150.3322, -78.4698)
  line L1363 (-157.6629, -73.6565) -> (-157.6167, -73.9203)
  line L1364 (-144.9025, -71.2185) -> (-144.93, -70.9336)
  line L1365 (-88.4902, -79.7153) -> (-88.3054, -79.7063)
  line L1366 (-154.9347, -77.6512) -> (-154.6713, -77.797)
  line L1367 (-115.1452, -70.2308) -> (-115.0907, -70.0127)
  line L1368 (-115.8241, -71.4744) -> (-115.6974, -71.3251)
  line L1369 (-115.6974, -71.3251) -> (-115.5801, -71.1668)
  line L1370 (-102.2516, -65.7009) -> (-102.3649, -65.6702)
  line L1371 (-56.2833, -68.7288) -> (-56.1225, -68.7825)
  line L1372 (-116.3544, -66.3241) -> (-116.5003, -66.219)
  line L1373 (-121.357, -72.3274) -> (-121.2734, -72.482)
  line L1374 (-121.4203, -72.1465) -> (-121.357, -72.3274)
  line L1375 (-121.3161, -71.3013) -> (-121.3776, -71.4014)
  line L1376 (-115.9599, -71.6151) -> (-115.8241, -71.4744)
  line L1377 (-134.4133, -81.6953) -> (-134.3896, -81.8899)
  line L1378 (-147.0665, -77.0991) -> (-146.8374, -76.8954)
  line L1379 (-121.3776, -71.4014) -> (-121.4259, -71.5165)
  line L1380 (-114.9978, -68.8249) -> (-115.0145, -68.6272)
  line L1381 (-146.4149, -76.4518) -> (-146.2219, -76.2125)
  line L1382 (-146.2219, -76.2125) -> (-146.0412, -75.9619)
  line L1383 (-149.9816, -78.4158) -> (-149.6412, -78.3469)
  line L1384 (-147.0666, -66.8727) -> (-147.3173, -66.6831)
  line L1385 (-145.4448, -74.8511) -> (-145.328, -74.5476)
  line L1386 (-145.328, -74.5476) -> (-145.2244, -74.2342)
  line L1387 (-146.2105, -67.7326) -> (-146.403, -67.5037)
  line L1388 (-146.0412, -75.9619) -> (-145.873, -75.7002)
  line L1389 (-123.6866, -67.3062) -> (-123.7123, -67.1111)
  line L1390 (-123.7123, -67.1111) -> (-123.7502, -66.9213)
  line L1391 (-123.1539, -66.9883) -> (-123.4156, -67.2357)
  line L1392 (-123.4156, -67.2357) -> (-123.6722, -67.5054)
  line L1393 (-121.1733, -65.8221) -> (-121.4727, -65.9327)
  line L1394 (-121.7664, -66.0609) -> (-122.0547, -66.2072)
  line L1395 (-121.4727, -65.9327) -> (-121.7664, -66.0609)
  line L1396 (-120.2412, -65.589) -> (-120.5577, -65.6509)
  line L1397 (-145.5747, -75.1445) -> (-145.4448, -74.8511)
  line L1398 (-122.0547, -66.2072) -> (-122.3375, -66.3725)
  line L1399 (-126.9445, -68.6517) -> (-126.9332, -68.8866)
  line L1400 (-123.8658, -66.5621) -> (-123.9451, -66.3953)
  line L1401 (-124.772, -65.6493) -> (-124.9758, -65.5788)
  line L1402 (-145.5783, -68.7237) -> (-145.7161, -68.4659)
  line L1403 (-145.7161, -68.4659) -> (-145.8673, -68.2144)
  line L1404 (-145.0573, -73.5791) -> (-144.9942, -73.2378)
  line L1405 (-144.9942, -73.2378) -> (-144.9448, -72.8877)
  line L1406 (-127.1731, -67.4104) -> (-127.1076, -67.6416)
  line L1407 (-155.9608, -71.3588) -> (-156.201, -71.3588)
  line L1408 (-150.8102, -71.3588) -> (-150.9298, -71.3363)
  line L1409 (-155.7174, -71.3283) -> (-155.841, -71.3363)
  line L1410 (-127.2532, -66.5328) -> (-127.278, -66.671)
  line L1411 (-127.286, -66.8152) -> (-127.2707, -67.0128)
  line L1412 (-127.278, -66.671) -> (-127.286, -66.8152)
  line L1413 (-145.2244, -74.2342) -> (-145.1341, -73.9113)
  line L1414 (-127.0421, -67.9152) -> (-126.9849, -68.2467)
  line L1415 (-126.9621, -68.439) -> (-126.9445, -68.6517)
  line L1416 (-156.4103, -71.3628) -> (-156.6012, -71.3747)
  line L1417 (-157.195, -71.5197) -> (-157.3044, -71.5845)
  line L1418 (-127.0901, -66.1588) -> (-127.1583, -66.2762)
  line L1419 (-157.0707, -71.4672) -> (-157.195, -71.5197)
  line L1420 (-144.9689, -70.6491) -> (-145.0194, -70.3657)
  line L1421 (-145.0194, -70.3657) -> (-145.0817, -70.0839)
  line L1422 (-144.9094, -72.529) -> (-144.8881, -72.1621)
  line L1423 (-144.8881, -72.1621) -> (-144.8811, -71.7871)
  line L1424 (-155.4279, -77.3274) -> (-155.1869, -77.4945)
  line L1425 (-155.1869, -77.4945) -> (-154.9347, -77.6512)
  line L1426 (-155.8755, -76.964) -> (-155.6574, -77.1504)
  line L1427 (-155.6574, -77.1504) -> (-155.4279, -77.3274)
  line L1428 (-90.0756, -81.8768) -> (-90.103, -81.6973)
  line L1429 (-157.4009, -74.6967) -> (-157.3035, -74.9488)
  line L1430 (-157.1936, -75.1965) -> (-157.0712, -75.4395)
  line L1431 (-157.3035, -74.9488) -> (-157.1936, -75.1965)
  line L1432 (-157.6167, -73.9203) -> (-157.5576, -74.182)
  line L1433 (-154.6713, -77.797) -> (-154.3968, -77.9313)
  line L1434 (-152.5229, -78.4681) -> (-152.1737, -78.5079)
  line L1435 (-156.9366, -75.6773) -> (-156.7897, -75.9092)
  line L1436 (-152.8617, -78.4132) -> (-152.5229, -78.4681)
  line L1437 (-144.8811, -71.7871) -> (-144.8861, -71.5032)
  line L1438 (-144.8861, -71.5032) -> (-144.9025, -71.2185)
  line L1439 (-145.873, -75.7002) -> (-145.7175, -75.4276)
  line L1440 (-148.9921, -78.1655) -> (-148.6836, -78.0535)
  line L1441 (-148.386, -77.9276) -> (-148.0994, -77.7881)
  line L1442 (-148.6836, -78.0535) -> (-148.386, -77.9276)
  line L1443 (-150.3322, -78.4698) -> (-149.9816, -78.4158)
  line L1444 (-147.3173, -66.6831) -> (-147.583, -66.5049)
  line L1445 (-146.403, -67.5037) -> (-146.6097, -67.2837)
  line L1446 (-144.9448, -72.8877) -> (-144.9094, -72.529)
  line L1447 (-145.1561, -69.8046) -> (-145.2427, -69.5282)
  line L1448 (-145.2427, -69.5282) -> (-145.3418, -69.2555)
  line L1449 (-149.3113, -78.2634) -> (-148.9921, -78.1655)
  line L1450 (-118.406, -72.7853) -> (-117.9611, -72.6722)
  line L1451 (-145.0817, -70.0839) -> (-145.1561, -69.8046)
  line L1452 (-117.9611, -72.6722) -> (-117.5374, -72.5382)
  line L1453 (-119.354, -70.5472) -> (-119.5376, -70.6259)
  line L1454 (-116.0791, -66.5536) -> (-116.2139, -66.4357)
  line L1455 (-119.7376, -70.6965) -> (-119.9539, -70.7594)
  line L1456 (-115.8284, -66.8085) -> (-115.9505, -66.6779)
  line L1457 (-120.1863, -70.8151) -> (-120.4347, -70.8642)
  line L1458 (-115.6051, -67.0878) -> (-115.7132, -66.9451)
  line L1459 (-120.6989, -70.9072) -> (-120.7434, -70.9215)
  line L1460 (-115.412, -67.3908) -> (-115.5046, -67.2364)
  line L1461 (-120.8538, -70.9601) -> (-121.0036, -71.031)
  line L1462 (-115.2518, -67.7168) -> (-115.3276, -67.551)
  line L1463 (-121.0851, -71.081) -> (-121.1665, -71.1421)
  line L1464 (-115.1275, -68.065) -> (-115.185, -67.8882)
  line L1465 (-121.2446, -71.2152) -> (-121.3161, -71.3013)
  line L1466 (-115.0419, -68.4346) -> (-115.0797, -68.2472)
  line L1467 (-123.7502, -66.9213) -> (-123.8011, -66.7379)
  line L1468 (-123.8011, -66.7379) -> (-123.8658, -66.5621)
  line L1469 (-56.986, -68.5784) -> (-56.6229, -68.6408)
  line L1470 (-148.4729, -66.0456) -> (-148.8011, -65.9197)
  line L1471 (-147.864, -66.3389) -> (-148.1606, -66.1855)
  line L1472 (-147.583, -66.5049) -> (-147.864, -66.3389)
  line L1473 (-156.1262, -68.728) -> (-155.9982, -68.7684)
  line L1474 (-149.5063, -65.7125) -> (-149.8837, -65.6326)
  line L1475 (-149.1455, -65.8084) -> (-149.5063, -65.7125)
  line L1476 (-148.8011, -65.9197) -> (-149.1455, -65.8084)
  line L1477 (-155.9982, -68.7684) -> (-155.8602, -68.7958)
  line L1478 (-155.5538, -68.8063) -> (-155.3855, -68.7888)
  line L1479 (-155.8602, -68.7958) -> (-155.712, -68.8093)
  line L1480 (-155.712, -68.8093) -> (-155.5538, -68.8063)
  line L1481 (-148.1606, -66.1855) -> (-148.4729, -66.0456)
  line L1482 (-60.3899, -69.3433) -> (-60.2729, -69.243)
  line L1483 (-60.2729, -69.243) -> (-60.1495, -69.1495)
  line L1484 (-148.4134, -73.094) -> (-148.4494, -73.3107)
  line L1485 (-151.1178, -65.4952) -> (-151.5638, -65.4852)
  line L1486 (-153.0467, -75.6737) -> (-153.26, -75.5238)
  line L1487 (-150.6892, -65.5233) -> (-151.1178, -65.4952)
  line L1488 (-153.26, -75.5238) -> (-153.4589, -75.3547)
  line L1489 (-148.8362, -69.5514) -> (-148.7604, -69.6794)
  line L1490 (-151.1946, -68.2097) -> (-151.0175, -68.2287)
  line L1491 (-151.5688, -68.2021) -> (-151.5638, -68.1941)
  line L1492 (-151.5638, -68.1941) -> (-151.3767, -68.1981)
  line L1493 (-156.6152, -68.3649) -> (-156.5375, -68.4558)
  line L1494 (-150.278, -65.5693) -> (-150.6892, -65.5233)
  line L1495 (-148.4494, -73.3107) -> (-148.4944, -73.5307)
  line L1496 (-153.4589, -75.3547) -> (-153.6426, -75.1674)
  line L1497 (-149.0063, -69.31) -> (-148.9182, -69.4283)
  line L1498 (-148.9182, -69.4283) -> (-148.8362, -69.5514)
  line L1499 (-149.8837, -65.6326) -> (-150.278, -65.5693)
  line L1500 (-153.6426, -75.1674) -> (-153.8102, -74.963)
  line L1501 (-149.2005, -69.0888) -> (-149.1004, -69.1968)
  line L1502 (-156.8418, -67.2086) -> (-156.8702, -67.3645)
  line L1503 (-151.5638, -65.4852) -> (-155.3858, -66.0126)
  line L1504 (-152.82, -75.8033) -> (-153.0467, -75.6737)
  line L1505 (-148.6277, -69.9489) -> (-148.5709, -70.0901)
  line L1506 (-155.6879, -66.0892) -> (-155.8344, -66.143)
  line L1507 (-152.068, -76.0606) -> (-152.3297, -75.9978)
  line L1508 (-155.3858, -66.0126) -> (-155.538, -66.0457)
  line L1509 (-152.5807, -75.9117) -> (-152.82, -75.8033)
  line L1510 (-149.7887, -68.6325) -> (-149.6596, -68.7121)
  line L1511 (-149.6596, -68.7121) -> (-149.5362, -68.7977)
  line L1512 (-148.5709, -70.0901) -> (-148.4766, -70.385)
  line L1513 (-155.9761, -66.2068) -> (-156.112, -66.2805)
  line L1514 (-156.112, -66.2805) -> (-156.2408, -66.364)
  line L1515 (-151.1789, -76.0985) -> (-151.5156, -76.112)
  line L1516 (-150.3604, -68.3768) -> (-150.2093, -68.431)
  line L1517 (-155.538, -66.0457) -> (-155.6879, -66.0892)
  line L1518 (-152.3297, -75.9978) -> (-152.5807, -75.9117)
  line L1519 (-148.7604, -69.6794) -> (-148.6909, -69.8119)
  line L1520 (-148.6909, -69.8119) -> (-148.6277, -69.9489)
  line L1521 (-155.3855, -68.7888) -> (-151.5688, -68.2021)
  line L1522 (-155.8344, -66.143) -> (-155.9761, -66.2068)
  line L1523 (-151.7963, -76.099) -> (-152.068, -76.0606)
  line L1524 (-149.4185, -68.8891) -> (-149.3066, -68.9862)
  line L1525 (-149.3066, -68.9862) -> (-149.2005, -69.0888)
  line L1526 (-149.9234, -68.559) -> (-149.7887, -68.6325)
  line L1527 (-156.5724, -66.6715) -> (-156.6607, -66.7925)
  line L1528 (-150.067, -75.8029) -> (-150.3116, -75.9096)
  line L1529 (-149.5362, -68.7977) -> (-149.4185, -68.8891)
  line L1530 (-151.5156, -76.112) -> (-151.7963, -76.099)
  line L1531 (-156.3612, -66.4571) -> (-156.4722, -66.5597)
  line L1532 (-150.5778, -75.9956) -> (-150.8666, -76.0591)
  line L1533 (-148.4086, -70.6952) -> (-148.3674, -71.0195)
  line L1534 (-148.3376, -71.8133) -> (-148.3368, -72.1199)
  line L1535 (-149.2876, -75.2032) -> (-149.4545, -75.3756)
  line L1536 (-156.7358, -66.9224) -> (-156.7966, -67.0611)
  line L1537 (-149.6394, -75.5342) -> (-149.8433, -75.6772)
  line L1538 (-151.0175, -68.2287) -> (-150.8454, -68.2552)
  line L1539 (-150.8454, -68.2552) -> (-150.6785, -68.2887)
  line L1540 (-148.4766, -70.385) -> (-148.4086, -70.6952)
  line L1541 (-149.1004, -69.1968) -> (-149.0063, -69.31)
  line L1542 (-148.6151, -73.9737) -> (-148.6926, -74.1932)
  line L1543 (-156.8539, -67.8212) -> (-156.8261, -67.9386)
  line L1544 (-148.7827, -74.4092) -> (-148.8863, -74.6199)
  line L1545 (-156.8807, -67.5289) -> (-156.8717, -67.7015)
  line L1546 (-149.0044, -74.8237) -> (-149.1379, -75.0187)
  line L1547 (-148.3674, -71.0195) -> (-148.3536, -71.3569)
  line L1548 (-148.3855, -72.8823) -> (-148.4134, -73.094)
  line L1549 (-156.6829, -68.2667) -> (-156.6152, -68.3649)
  line L1550 (-148.4944, -73.5307) -> (-148.5493, -73.7522)
  line L1551 (-153.8102, -74.963) -> (-153.9608, -74.7424)
  line L1552 (-153.9608, -74.7424) -> (-154.0934, -74.5067)
  line L1553 (-154.2073, -74.2569) -> (-154.3015, -73.9941)
  line L1554 (-154.0934, -74.5067) -> (-154.2073, -74.2569)
  line L1555 (-60.6041, -69.5643) -> (-60.5003, -69.4503)
  line L1556 (-150.4755, -71.5011) -> (-150.6265, -71.419)
  line L1557 (-151.0517, -73.4333) -> (-150.9441, -73.4273)
  line L1558 (-150.6418, -73.35) -> (-150.5497, -73.3056)
  line L1559 (-150.6265, -71.419) -> (-150.7911, -71.3619)
  line L1560 (-154.3752, -73.7192) -> (-154.4274, -73.4333)
  line L1561 (-150.0587, -72.0296) -> (-150.1296, -71.8724)
  line L1562 (-150.1296, -71.8724) -> (-150.2244, -71.7303)
  line L1563 (-149.9987, -72.3794) -> (-150.0027, -72.2883)
  line L1564 (-150.0027, -72.2883) -> (-150.0142, -72.1994)
  line L1565 (-154.3015, -73.9941) -> (-154.3752, -73.7192)
  line L1566 (-150.0457, -72.6924) -> (-150.0197, -72.5915)
  line L1567 (-154.4274, -73.4333) -> (-151.0517, -73.4333)
  line L1568 (-150.7386, -73.3855) -> (-150.6418, -73.35)
  line L1569 (-150.7911, -71.3619) -> (-150.7901, -71.3559)
  line L1570 (-150.0142, -72.1994) -> (-150.0587, -72.0296)
  line L1571 (-150.1783, -72.9682) -> (-150.1255, -72.8813)
  line L1572 (-150.9441, -73.4273) -> (-150.8395, -73.4114)
  line L1573 (-150.239, -73.0493) -> (-150.1783, -72.9682)
  line L1574 (-61.1878, -70.7284) -> (-61.1395, -70.5579)
  line L1575 (-60.7012, -69.6851) -> (-60.6041, -69.5643)
  line L1576 (-60.8751, -69.9478) -> (-60.7916, -69.813)
  line L1577 (-151.3767, -68.1981) -> (-151.1946, -68.2097)
  line L1578 (-148.3536, -71.3569) -> (-148.3456, -71.5748)
  line L1579 (-148.3456, -71.5748) -> (-148.3376, -71.8133)
  line L1580 (-60.1495, -69.1495) -> (-60.0196, -69.0628)
  line L1581 (-156.2441, -68.6756) -> (-156.1262, -68.728)
  line L1582 (-156.3519, -68.6121) -> (-156.2441, -68.6756)
  line L1583 (-156.7883, -68.0526) -> (-156.7406, -68.1623)
  line L1584 (-156.7406, -68.1623) -> (-156.6829, -68.2667)
  line L1585 (-148.5493, -73.7522) -> (-148.6151, -73.9737)
  line L1586 (-150.1255, -72.8813) -> (-150.0811, -72.7892)
  line L1587 (-150.0811, -72.7892) -> (-150.0457, -72.6924)
  line L1588 (-150.0197, -72.5915) -> (-150.0037, -72.487)
  line L1589 (-150.0037, -72.487) -> (-149.9987, -72.3794)
  line L1590 (-60.5003, -69.4503) -> (-60.3899, -69.3433)
  line L1591 (-150.5497, -73.3056) -> (-150.4629, -73.2528)
  line L1592 (-150.3818, -73.1921) -> (-150.307, -73.1241)
  line L1593 (-150.4629, -73.2528) -> (-150.3818, -73.1921)
  line L1594 (-150.8395, -73.4114) -> (-150.7386, -73.3855)
  line L1595 (-150.307, -73.1241) -> (-150.239, -73.0493)
  line L1596 (-150.7901, -71.3559) -> (-150.8102, -71.3588)
  line L1597 (-150.6785, -68.2887) -> (-150.5168, -68.3293)
  line L1598 (-150.5168, -68.3293) -> (-150.3604, -68.3768)
  line L1599 (-156.2408, -66.364) -> (-156.3612, -66.4571)
  line L1600 (-150.8666, -76.0591) -> (-151.1789, -76.0985)
  line L1601 (-156.4722, -66.5597) -> (-156.5724, -66.6715)
  line L1602 (-150.3116, -75.9096) -> (-150.5778, -75.9956)
  line L1603 (-156.6607, -66.7925) -> (-156.7358, -66.9224)
  line L1604 (-149.8433, -75.6772) -> (-150.067, -75.8029)
  line L1605 (-156.7966, -67.0611) -> (-156.8418, -67.2086)
  line L1606 (-149.4545, -75.3756) -> (-149.6394, -75.5342)
  line L1607 (-156.8702, -67.3645) -> (-156.8807, -67.5289)
  line L1608 (-149.1379, -75.0187) -> (-149.2876, -75.2032)
  line L1609 (-156.8717, -67.7015) -> (-156.8539, -67.8212)
  line L1610 (-148.8863, -74.6199) -> (-149.0044, -74.8237)
  line L1611 (-156.8261, -67.9386) -> (-156.7883, -68.0526)
  line L1612 (-148.6926, -74.1932) -> (-148.7827, -74.4092)
  line L1613 (-150.2244, -71.7303) -> (-150.3406, -71.6057)
  line L1614 (-150.3406, -71.6057) -> (-150.4755, -71.5011)
  line L1615 (-61.4018, -81.887) -> (-61.3587, -81.6928)
  line L1616 (-61.8529, -82.6864) -> (-61.7328, -82.5514)
  line L1617 (-61.3081, -71.4835) -> (-61.2891, -71.2837)
  line L1618 (-61.3235, -71.9056) -> (-61.3195, -71.6908)
  line L1619 (-61.3195, -71.6908) -> (-61.3081, -71.4835)
  line L1620 (-142.4212, -66.1208) -> (-142.5144, -66.252)
  line L1621 (-142.7784, -67.3778) -> (-142.7498, -67.5649)
  line L1622 (-142.7566, -66.8474) -> (-142.7808, -67.0086)
  line L1623 (-142.7073, -67.7335) -> (-142.6551, -67.8835)
  line L1624 (-142.7888, -67.1725) -> (-142.7784, -67.3778)
  line L1625 (-134.3896, -81.8899) -> (-134.3507, -82.0716)
  line L1626 (-142.7498, -67.5649) -> (-142.7073, -67.7335)
  line L1627 (-140.9924, -65.4901) -> (-141.1482, -65.4851)
  line L1628 (-140.3446, -65.6405) -> (-140.4577, -65.5959)
  line L1629 (-141.644, -65.5652) -> (-141.7958, -65.6248)
  line L1630 (-86.8381, -66.1295) -> (-86.7617, -66.2638)
  line L1631 (-46.9857, -80.9562) -> (-47.0979, -80.9274)
  line L1632 (-101.4961, -66.1748) -> (-101.5617, -66.1074)
  line L1633 (-89.912, -66.407) -> (-89.8498, -66.2638)
  line L1634 (-112.5708, -66.858) -> (-112.6041, -67.0202)
  line L1635 (-95.8703, -66.1296) -> (-95.9551, -66.2307)
  line L1636 (-46.7759, -81.0448) -> (-46.8782, -80.9955)
  line L1637 (-88.3054, -83.3197) -> (-88.4902, -83.3107)
  line L1638 (-90.037, -67.0481) -> (-90.0226, -66.8796)
  line L1639 (-87.842, -78.5031) -> (-88.063, -78.5303)
  line L1640 (-90.103, -81.3276) -> (-90.0756, -81.1482)
  line L1641 (-69.2394, -83.2381) -> (-69.1231, -83.2204)
  line L1642 (-96.1626, -66.5764) -> (-96.2143, -66.7049)
  line L1643 (-112.6072, -67.5226) -> (-112.5744, -67.6917)
  line L1644 (-47.2141, -80.9097) -> (-47.3337, -80.9037)
  line L1645 (-96.0325, -66.3391) -> (-96.1018, -66.4544)
  line L1646 (-90.0311, -80.975) -> (-89.9704, -80.809)
  line L1647 (-47.3337, -80.9037) -> (-50.3366, -80.9037)
  line L1648 (-88.5487, -78.5303) -> (-88.7696, -78.5031)
  line L1649 (-68.9034, -83.1522) -> (-68.801, -83.1029)
  line L1650 (-90.0226, -66.8796) -> (-89.9976, -66.7159)
  line L1651 (-90.0226, -77.145) -> (-90.037, -76.9765)
  line L1652 (-88.3059, -78.5393) -> (-88.5487, -78.5303)
  line L1653 (-89.3159, -83.0114) -> (-89.4549, -82.9073)
  line L1654 (-89.6998, -82.6623) -> (-89.8038, -82.5231)
  line L1655 (-46.8782, -80.9955) -> (-46.9857, -80.9562)
  line L1656 (-112.6041, -67.0202) -> (-112.6217, -67.1857)
  line L1657 (-199, -135) -> (-151, -135)
  line L1658 (-150, -136) -> (-150, -164)
  arc A7 (-200, -134) -> (-199, -135) centre (-199, -134) ccw
  arc A8 (-150, -136) -> (-151, -135) centre (-151, -136) ccw
  arc A9 (-150, -164) -> (-149, -165) centre (-149, -164) ccw